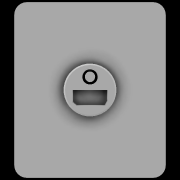
# Autodesk Inventor part: fishman-battery
Saved by Autodesk Inventor 2020 (Build 240168000, 168)
## iProperties
Created: 2020-01-01
Part Number: fishman-battery
Material: Generic
Document SubType Name: Modeling
Designer: valer
Density: 1 g/cm^3
Appearance: Default
Author: valer
Autodesk Inventor part; units mm, degrees
ref_plane "YZ Plane" through (0, 0, 0) normal (1, 0, 0) x (0, 1, 0)
ref_plane "XZ Plane" through (0, 0, 0) normal (0, 1, 0) x (-1, 0, 0)
ref_plane "XY Plane" through (0, 0, 0) normal (0, 0, 1) x (1, 0, 0)
sketch "FishmanBattery" plane through (0, 0, 0) normal (0, 0, 1) x (1, 0, 0)
  line L0 (-19.05, 22.098) -> (19.05, 22.098)
  line L1 (19.05, 22.098) -> (19.05, -22.098)
  line L2 (19.05, -22.098) -> (-19.05, -22.098)
  line L3 (-19.05, -22.098) -> (-19.05, 22.098)
  circle A0 centre (0, 0) radius 6.35
  line L4 (0, 22.098) -> (0, -22.098) construction
  line L5 (-19.05, 0) -> (19.05, 0) construction
  point P0 (0, 0)
  point P1 (0, 0)
  dimension "d13" = 38.1
  dimension "d14" = 44.196
  dimension "d26" = 12.7
  constraints: 12 end point, 6 midpoint, 2 coincident, 2 parallel, 1 centre point, 1 horizontal, 1 perpendicular
  measures "d13" distance of L0.start L0.end
  measures "d14" distance of L2.end L0.start
  measures "d26" diameter of A0
extrude "FishmanBatteryFeature" add sketch "FishmanBattery" against normal blind 10.16 contours L0 L1 L2 L3 | A0
extrude "FishmanBatteryConnectorFeature" add sketch "FishmanBattery" along normal blind 3.81 contours A0
chamfer "FishmanBatteryChamferFeature" distance 0.381 angle 45 1 edges at (-6.35, 0, 3.81)
fillet "FishmanBatteryFilletsFeature" radius 3.175 4 edges at (19.05, 22.098, -5.08) (19.05, -22.098, -5.08) (-19.05, -22.098, -5.08) (-19.05, 22.098, -5.08)
sketch "FishmanConnector" plane through (0, 0, 3.81) normal (0, 0, 1) x (1, 0, 0)
  circle A0 centre (0, 3.175) radius 1.8791
  circle A1 centre (0, 3.175) radius 1.2441
  line L0 (-4.2333, 0) -> (4.2333, 0)
  line L1 (4.2333, 0) -> (4.2333, -2.6291)
  line L2 (4.2333, -2.6291) -> (3.5983, -3.729)
  line L3 (3.5983, -3.729) -> (-3.2605, -3.729)
  line L4 (-3.2605, -3.729) -> (-4.2333, -2.9126)
  line L5 (-4.2333, -2.9126) -> (-4.2333, 0)
  line L6 (0, -30.9372) -> (0, 30.9372) construction
  point P0 (0, 0)
  point P1 (0, 0)
  dimension "d133" = 3.729
  dimension "d134" = 8.4667
  dimension "d135" = 3.7582
  dimension "d136" = 0.635
  dimension "d137" = 150
  dimension "d138" = 140
  dimension "d139" = 1.27
  dimension "d141" = 3.175
  constraints: 12 end point, 3 midpoint, 2 centre point, 2 parallel, 2 perpendicular, 1 coincident, 1 equal length, 1 point on line
  measures "d133" distance between parallel lines of L0 L3
  measures "d134" distance of L0.start L0.end
  measures "d135" diameter of A0
  measures "d136" radial gap between concentric circles of A0 A1
  measures "d137" angle of L2 L1
  measures "d138" angle of L3 L4
  measures "d139" distance of L3.end L4.end
  measures "d141" distance from line of L0 A0.centre
extrude "FishmanConnectorHolesFeature" cut sketch "FishmanConnector" against normal blind 3.81
body "Solid3"
